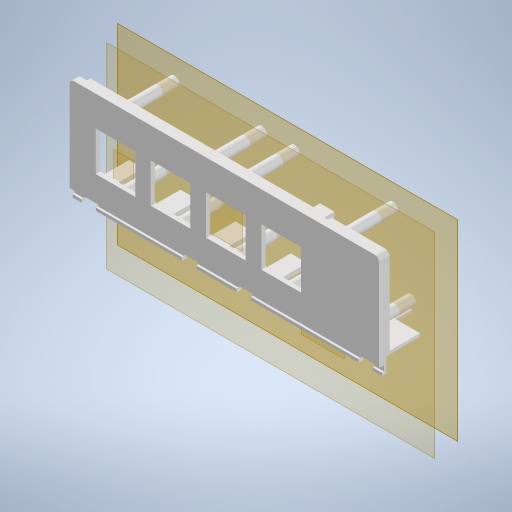
# Autodesk Inventor part: RV_ES_TopHV
Saved by Autodesk Inventor 2023.3 (Build 273359000, 359)
## iProperties
Created: 2023-08-06
Part Number: RV_ES_TopHV
Material: Generic
Document SubType Name: Modeling
Designer: atrus
Density: 1 g/cm^3
Appearance: Default
Mass: 78.5507 g
Surface Area: 462.891 cm^2
Volume: 78.5507 cm^3
Author: atrus
Autodesk Inventor part; units mm, degrees
ref_plane "YZ Plane" through (0, 0, 0) normal (1, 0, 0) x (0, 1, 0)
ref_plane "XZ Plane" through (0, 0, 0) normal (0, 1, 0) x (-1, 0, 0)
ref_plane "XY Plane" through (0, 0, 0) normal (0, 0, 1) x (1, 0, 0)
ref_plane "Work Plane1" through (160.7185, -7.942384, -39.091557) normal (0, 0, 1) x (1, 0, 0)
ref_plane "Bottom Case Offset" through (160.7185, -7.942384, -38.891557) normal (0, 0, 1) x (1, 0, 0)
sketch "Sketch1" plane through (0, 0, 0) normal (0, 0, 1) x (1, 0, 0)
  line L0 (0, 55.614096) -> (215.9, 55.614096)
  line L1 (215.9, 55.614096) -> (215.9, 121.724616)
  line L2 (215.9, 121.724616) -> (0, 121.724616)
  line L3 (0, 121.724616) -> (0, 55.614096)
  line L4 (215.9, 121.724616) -> (215.9, 57.656276) construction
  line L5 (0, 48.884616) -> (0, 118.549616)
  line L6 (1.113, 48.884616) -> (0, 48.884616)
  point P0 (0, 88.669356)
  constraints: 10 end point, 2 parallel, 1 horizontal, 1 midpoint, 1 perpendicular
extrude "Top Face" add sketch "Sketch1" along normal blind 5
sketch "Sketch2" plane through (0, 0, 5) normal (0, 0, 1) x (1, 0, 0)
  line L0 (44.754719, 74.175735) -> (19.253119, 74.175735) construction
  line L1 (44.754719, 99.677335) -> (44.754719, 74.175735) construction
  line L2 (19.253119, 74.175735) -> (19.253119, 99.677335) construction
  line L3 (57.607119, 74.175735) -> (57.607119, 99.677335) construction
  line L4 (83.108719, 99.677335) -> (83.108719, 74.175735) construction
  line L5 (83.108719, 74.175735) -> (57.607119, 74.175735) construction
  line L6 (96.215119, 74.175735) -> (96.215119, 99.677335) construction
  line L7 (121.716719, 99.677335) -> (121.716719, 74.175735) construction
  line L8 (134.823119, 74.175735) -> (134.823119, 99.677335) construction
  line L9 (160.324719, 99.677335) -> (160.324719, 74.175735) construction
  line L10 (160.324719, 74.175735) -> (134.823119, 74.175735) construction
  line L11 (19.253119, 99.677335) -> (44.754719, 99.677335) construction
  line L12 (57.607119, 99.677335) -> (83.108719, 99.677335) construction
  line L13 (96.215119, 99.677335) -> (121.716719, 99.677335) construction
  line L14 (134.823119, 99.677335) -> (160.324719, 99.677335) construction
  line L15 (18.253119, 100.677335) -> (18.253119, 73.175735)
  line L16 (18.253119, 73.175735) -> (45.754719, 73.175735)
  line L17 (45.754719, 73.175735) -> (45.754719, 100.677335)
  line L18 (45.754719, 100.677335) -> (18.253119, 100.677335)
  line L19 (56.607119, 100.677335) -> (56.607119, 73.175735)
  line L20 (56.607119, 73.175735) -> (84.108719, 73.175735)
  line L21 (84.108719, 73.175735) -> (84.108719, 100.677335)
  line L22 (84.108719, 100.677335) -> (56.607119, 100.677335)
  line L23 (121.716719, 74.175735) -> (96.215119, 74.175735) construction
  line L24 (96.215119, 74.175735) -> (96.215119, 99.677335)
  line L25 (95.215119, 100.677335) -> (95.215119, 73.175735)
  line L26 (95.215119, 73.175735) -> (122.716719, 73.175735)
  line L27 (122.716719, 73.175735) -> (122.716719, 100.677335)
  line L28 (122.716719, 100.677335) -> (95.215119, 100.677335)
  line L29 (133.823119, 100.677335) -> (133.823119, 73.175735)
  line L30 (133.823119, 73.175735) -> (161.324719, 73.175735)
  line L31 (161.324719, 73.175735) -> (161.324719, 100.677335)
  line L32 (161.324719, 100.677335) -> (133.823119, 100.677335)
  point P0 (0, 0)
  dimension "d96" = 1
  constraints: 32 end point, 3 parallel, 12 other
  measures "d96" distance between parallel lines of L18 L11
extrude "Recept Cutouts" cut sketch "Sketch2" against normal blind 3
sketch "Sketch3" plane through (0, 0, 0) normal (0, 0, -1) x (-1, 0, 0)
  circle A0 centre (-90.17, 112.834616) radius 3.750005 construction
  circle A1 centre (-181.61, 112.834616) radius 3.750005 construction
  circle A2 centre (-29.21, 112.834616) radius 3.550005
  circle A3 centre (-32.004, 65.844616) radius 3.550005
  circle A4 centre (-70.358, 65.844616) radius 3.550005
  circle A5 centre (-90.17, 112.834616) radius 3.550005
  circle A6 centre (-113.03, 112.834616) radius 3.550005
  circle A7 centre (-108.966, 65.844616) radius 3.550005
  circle A8 centre (-181.61, 112.834616) radius 3.550005
  circle A9 centre (-194.31, 63.304616) radius 3.550005
  circle A10 centre (-29.21, 112.834616) radius 3.81
  circle A11 centre (-32.004, 65.844616) radius 3.81
  circle A12 centre (-113.03, 112.834616) radius 3.81
  circle A13 centre (-70.358, 65.844616) radius 3.81
  circle A14 centre (-108.966, 65.844616) radius 3.81
  circle A15 centre (-194.31, 63.304616) radius 3.81
  circle A16 centre (-147.574, 65.844616) radius 3.750005
  circle A17 centre (-147.574, 65.844616) radius 3.550005
  point P0 (0, 0)
  dimension "d5" = 0.2
  constraints: 9 centre point, 8 equal radius, 7 coincident
  measures "d5" radial gap between concentric circles of A1 A8
extrude "Bosses" add sketch "Sketch3" along normal up to surface (38.891557 mm away) contours A2 | A3 | A4 | A5 | A6 | A7 | A8 | A9 | A17
ref_plane "PCB Plane Offset" through (103.01683, 55.15644, -27.328797) normal (0, 0, 1) x (1, 0, 0)
sketch "Sketch4" plane through (0, 0, 0) normal (0, 0, -1) x (-1, 0, 0)
  line L0 (-188.196091, 44.678615) -> (-188.196091, 97.078617) construction
  line L1 (-188.696091, 55.614096) -> (-212.089995, 55.614096)
  line L2 (-212.089995, 55.614096) -> (-212.089995, 57.846616)
  line L3 (-212.089995, 57.846616) -> (-188.696091, 57.846616)
  line L4 (-188.696091, 57.846616) -> (-188.696091, 55.614096)
  line L5 (-172.95, 57.946616) -> (-195.35, 57.946616)
  line L6 (-212.08999, -4.005394) -> (-212.09, 115.374616)
  line L7 (0, 55.614096) -> (-215.9, 55.614096)
  point P0 (0, 0)
  dimension "d8" = 0.5
  dimension "d109" = 0.1
  constraints: 8 end point, 3 perpendicular, 1 collinear, 1 horizontal
  measures "d8" distance between parallel lines of L0 L4
  measures "d109" distance between parallel lines of L5 L3
extrude "PS Side Tall Barrier" add sketch "Sketch4" along normal up to surface (27.328797 mm away)
sketch "Sketch5" plane through (212.089995, 57.846616, -27.328797) normal (0, 0, -1) x (-1, 0, 0)
  line L0 (23.393904, 0) -> (23.393904, -2.23252)
  line L1 (23.393904, 0) -> (0, 0)
  line L2 (23.393904, -2.23252) -> (16.939975, -2.23252)
  line L3 (16.939975, -2.23252) -> (16.939975, 0)
  line L4 (16.939975, 0) -> (23.393904, 0)
  line L5 (23.393904, 0) -> (23.393904, -2.23252)
  point P0 (212.089995, -57.846616)
  point P1 (16.739975, -2.8)
  dimension "d13" = 0.2
  constraints: 8 end point, 2 parallel, 1 horizontal, 1 perpendicular, 1 point on line, 1 other
  measures "d13" horizontal distance of point (16.74, -2.8) L2.end
extrude "PS Side Tall Barrier PCB" add sketch "Sketch5" along normal up to surface (11.56276 mm away)
sketch "Sketch6" plane through (0, 0, 0) normal (0, 0, -1) x (-1, 0, 0)
  arc A0 (-212.725, 121.724616) -> (-215.9, 118.549616) centre (-212.725, 118.549616) ccw construction
  arc A1 (-210.312, 119.311616) -> (-213.487, 116.136616) centre (-210.312, 116.136616) ccw construction
  line L0 (-213.487, 50.884616) -> (-213.487, 116.136616) construction
  line L1 (-210.312, 119.311616) -> (-172.72, 119.311616) construction
  line L2 (-162.72, 119.311616) -> (-5.588, 119.311616) construction
  arc A2 (-2.413, 116.136616) -> (-5.588, 119.311616) centre (-5.588, 116.136616) ccw construction
  line L3 (-2.413, 58.624616) -> (-2.413, 50.884616) construction
  line L4 (-213.287, 58.146616) -> (-213.287, 116.136616)
  arc A3 (-210.312, 119.111616) -> (-213.287, 116.136616) centre (-210.312, 116.136616) ccw
  line L5 (-210.312, 119.111616) -> (-172.72, 119.111616)
  line L6 (-162.72, 119.111616) -> (-5.588, 119.111616)
  arc A4 (-2.613, 116.136616) -> (-5.588, 119.111616) centre (-5.588, 116.136616) ccw
  line L7 (-2.613, 116.136616) -> (-2.613, 61.064616)
  line L8 (-211.287, 58.146616) -> (-211.287, 116.136616)
  arc A5 (-210.312, 117.111616) -> (-211.287, 116.136616) centre (-210.312, 116.136616) ccw
  arc A6 (-4.613, 116.136616) -> (-5.588, 117.111616) centre (-5.588, 116.136616) ccw
  line L9 (-4.613, 116.136616) -> (-4.613, 61.064616)
  line L10 (-211.287, 58.146616) -> (-213.287, 58.146616)
  line L11 (-4.613, 61.064616) -> (-2.613, 61.064616)
  line L12 (-162.72, 119.111616) -> (-162.72, 117.111616)
  line L13 (-172.72, 117.111616) -> (-172.72, 119.111616)
  circle A7 centre (-181.61, 112.834616) radius 3.550005
  line L14 (-178.059995, 112.834616) -> (-178.059995, 117.111616)
  circle A8 centre (-113.03, 112.834616) radius 3.550005
  line L15 (-116.580005, 112.834616) -> (-116.580005, 117.111616)
  line L16 (-109.479995, 112.834616) -> (-109.479995, 117.111616)
  circle A9 centre (-90.17, 112.834616) radius 3.550005
  line L17 (-93.720005, 112.834616) -> (-93.720005, 117.111616)
  line L18 (-86.619995, 112.834616) -> (-86.619995, 117.111616)
  circle A10 centre (-29.21, 112.834616) radius 3.550005
  line L19 (-32.760005, 112.834616) -> (-32.760005, 117.111616)
  line L20 (-25.659995, 112.834616) -> (-25.659995, 117.111616)
  circle A11 centre (-181.61, 112.834616) radius 3.550005
  circle A12 centre (-113.03, 112.834616) radius 3.550005
  line L21 (-185.160005, 112.834616) -> (-185.160005, 117.111616)
  line L22 (-210.312, 117.111616) -> (-185.160005, 117.111616)
  line L23 (-178.059995, 117.111616) -> (-172.72, 117.111616)
  line L24 (-162.72, 117.111616) -> (-116.580005, 117.111616)
  line L25 (-109.479995, 117.111616) -> (-93.720005, 117.111616)
  line L26 (-86.619995, 117.111616) -> (-32.760005, 117.111616)
  line L27 (-25.659995, 117.111616) -> (-5.588, 117.111616)
  line L28 (-195.15002, 57.846616) -> (-212.089995, 57.846616)
  line L29 (-3.81001, 60.764616) -> (-8.88109, 60.764616) construction
  line L30 (-188.696091, 57.846616) -> (-195.15002, 57.846616) construction
  point P0 (-212.287, 58.146616)
  dimension "d59" = 0.2
  dimension "d60" = 0.2
  dimension "d62" = 2
  dimension "d113" = 2
  dimension "d114" = 0.3
  dimension "d115" = 0.3
  constraints: 48 end point, 24 perpendicular, 15 point on circle, 8 collinear, 7 tangent, 4 centre point, 3 vertical, 2 horizontal, 2 parallel, 1 midpoint, 8 other
  measures "d59" distance between parallel lines of L2 L6
  measures "d60" distance between parallel lines of L0 L4
  measures "d62" distance of L13.start L5.end
  measures "d113" distance between parallel lines of L8 L4
  measures "d114" distance between parallel lines of L29 L11
  measures "d115" distance from line of L30 point (-212.287, 58.147)
extrude "Inner Lip" add sketch "Sketch6" along normal blind 5 contours L4 A3 L5 L13 L23 L14 A7 L21 L22 A5 L8 L10 | L6 A4 L7 L11 L9 A6 L27 L20 A10 L19 L26 L18 A9 L17 L25 L16 A8 L15 L24 L12
sketch "Sketch7" plane through (181.61, 112.834616, -38.891557) normal (0, 0, -1) x (-1, 0, 0)
  circle A0 centre (0, 0) radius 3.550005
  circle A1 centre (68.58, 0) radius 3.550005
  circle A2 centre (91.44, 0) radius 3.550005
  circle A3 centre (152.4, 0) radius 3.550005
  circle A4 centre (149.606, -46.99) radius 3.550005
  circle A5 centre (111.252, -46.99) radius 3.550005
  circle A6 centre (72.644, -46.99) radius 3.550005
  circle A7 centre (-12.7, -49.53) radius 3.550005
  circle A8 centre (34.036, -46.99) radius 3.550005
  point P0 (181.61, -112.834616)
hole "Boss Holes" at (181.61, 112.834616, -38.891557) at (113.03, 112.834616, -38.891557) at (90.17, 112.834616, -38.891557) at (29.21, 112.834616, -38.891557) at (32.004, 65.844616, -38.891557) at (70.358, 65.844616, -38.891557) at (108.966, 65.844616, -38.891557) at (194.31, 63.304616, -38.891557) at (147.574, 65.844616, -38.891557) direction (0, 0, 1) diameter 2.15646 depth 12.7 tip angle 118 thread size "4-40 UNC" class "2B" standard "ANSI Unified Screw Threads"
sketch "Sketch8" plane through (0, 0, 0) normal (0, 0, -1) x (-1, 0, 0)
  line L0 (-162.72, 117.111616) -> (-162.72, 121.724616)
  line L1 (-215.9, 121.724616) -> (0, 121.724616)
  line L2 (-172.72, 117.111616) -> (-172.72, 121.724616)
  line L3 (-162.72, 117.111616) -> (-116.580005, 117.111616) construction
  line L4 (-172.72, 117.111616) -> (-162.72, 117.111616)
  line L5 (-178.059995, 117.111616) -> (-172.72, 117.111616)
  line L6 (-172.72, 117.111616) -> (-172.72, 119.111616)
  line L7 (-162.72, 119.111616) -> (-162.72, 117.111616)
  line L8 (-172.72, 121.724616) -> (-162.72, 121.724616)
  point P0 (0, 0)
  point P1 (-172.72, 118.111616)
  constraints: 8 end point, 3 collinear, 1 horizontal, 1 midpoint, 1 perpendicular, 1 point on line, 1 vertical
extrude "Cord Relief" add sketch "Sketch8" along normal blind 7
fillet "Boss Filets" radius 3.175 9 edges at (181.61, 109.2846, 0) (35.554, 65.8446, 0) (73.908, 65.8446, 0) (112.516, 65.8446, 0) (197.86, 63.3046, 0) (113.03, 109.2846, 0) (90.17, 109.2846, 0) (29.21, 109.2846, 0) (151.124, 65.8446, 0)
ref_plane "Relay Top" through (28.37801, 48.104546, -10.841317) normal (0, 0, 1) x (0, -1, 0)
ref_plane "PS Top" through (155.310019, 43.098635, -2.554097) normal (0, 0, 1) x (0, 1, 0)
ref_plane "Work Plane7" through (-216.350226, -15.116245, -29.091557) normal (0, 0, 1) x (1, -0.0000001, 0)
sketch "Sketch10" plane through (0, 0, 0) normal (0, 0, -1) x (-1, 0, 0)
  line L0 (-160.996089, 97.078617) -> (-160.996089, 44.678615) construction
  line L1 (-188.196091, 44.678615) -> (-188.196091, 97.078617) construction
  line L2 (-122.08008, 67.154546) -> (-134.78008, 67.154546) construction
  line L3 (-134.78008, 67.154546) -> (-134.78008, 96.154546) construction
  line L4 (-134.78008, 96.154546) -> (-122.08008, 96.154546) construction
  line L5 (-122.08008, 96.154546) -> (-122.08008, 67.154546) construction
  line L6 (-123.43008, 68.054546) -> (-133.43008, 68.054546) construction
  line L7 (-123.43008, 69.054546) -> (-123.43008, 68.054546) construction
  line L8 (-133.43008, 69.054546) -> (-123.43008, 69.054546) construction
  line L9 (-133.43008, 68.054546) -> (-133.43008, 69.054546) construction
  line L10 (-133.83008, 88.254546) -> (-133.83008, 84.654546) construction
  line L11 (-133.83008, 84.654546) -> (-123.03008, 84.654546) construction
  line L12 (-123.03008, 84.654546) -> (-123.03008, 88.254546) construction
  line L13 (-123.03008, 88.254546) -> (-133.83008, 88.254546) construction
  line L14 (-83.21808, 67.154556) -> (-95.91808, 67.154556) construction
  line L15 (-95.91808, 67.154556) -> (-95.91808, 96.154556) construction
  line L16 (-95.91808, 96.154556) -> (-83.21808, 96.154556) construction
  line L17 (-83.21808, 96.154556) -> (-83.21808, 67.154556) construction
  line L18 (-84.56808, 68.054556) -> (-94.56808, 68.054556) construction
  line L19 (-84.56808, 69.054556) -> (-84.56808, 68.054556) construction
  line L20 (-94.56808, 69.054556) -> (-84.56808, 69.054556) construction
  line L21 (-94.56808, 68.054556) -> (-94.56808, 69.054556) construction
  line L22 (-94.96808, 88.254556) -> (-94.96808, 84.654556) construction
  line L23 (-94.96808, 84.654556) -> (-84.16808, 84.654556) construction
  line L24 (-84.16808, 84.654556) -> (-84.16808, 88.254556) construction
  line L25 (-84.16808, 88.254556) -> (-94.96808, 88.254556) construction
  line L26 (-44.86408, 67.154546) -> (-57.56408, 67.154546) construction
  line L27 (-57.56408, 67.154546) -> (-57.56408, 96.154546) construction
  line L28 (-57.56408, 96.154546) -> (-44.86408, 96.154546) construction
  line L29 (-44.86408, 96.154546) -> (-44.86408, 67.154546) construction
  line L30 (-46.21408, 68.054546) -> (-56.21408, 68.054546) construction
  line L31 (-46.21408, 69.054546) -> (-46.21408, 68.054546) construction
  line L32 (-56.21408, 69.054546) -> (-46.21408, 69.054546) construction
  line L33 (-56.21408, 68.054546) -> (-56.21408, 69.054546) construction
  line L34 (-56.61408, 88.254546) -> (-56.61408, 84.654546) construction
  line L35 (-56.61408, 84.654546) -> (-45.81408, 84.654546) construction
  line L36 (-45.81408, 84.654546) -> (-45.81408, 88.254546) construction
  line L37 (-45.81408, 88.254546) -> (-56.61408, 88.254546) construction
  line L38 (-6.13608, 67.154546) -> (-18.83608, 67.154546) construction
  line L39 (-18.83608, 67.154546) -> (-18.83608, 96.154546) construction
  line L40 (-18.83608, 96.154546) -> (-6.13608, 96.154546) construction
  line L41 (-6.13608, 96.154546) -> (-6.13608, 67.154546) construction
  line L42 (-7.48608, 68.054546) -> (-17.48608, 68.054546) construction
  line L43 (-7.48608, 69.054546) -> (-7.48608, 68.054546) construction
  line L44 (-17.48608, 69.054546) -> (-7.48608, 69.054546) construction
  line L45 (-17.48608, 68.054546) -> (-17.48608, 69.054546) construction
  line L46 (-17.88608, 88.254546) -> (-17.88608, 84.654546) construction
  line L47 (-17.88608, 84.654546) -> (-7.08608, 84.654546) construction
  line L48 (-7.08608, 84.654546) -> (-7.08608, 88.254546) construction
  line L49 (-7.08608, 88.254546) -> (-17.88608, 88.254546) construction
  line L50 (-195.15002, 55.614096) -> (-188.696091, 55.614096)
  line L51 (-188.696091, 55.614096) -> (-188.696091, 57.846616)
  line L52 (-188.696091, 57.846616) -> (-195.15002, 57.846616)
  line L53 (-195.15002, 57.846616) -> (-195.15002, 55.614096)
  line L54 (0, 55.614096) -> (-215.9, 55.614096)
  line L55 (-188.696091, 57.846616) -> (-195.15002, 57.846616)
  arc A0 (-43.204, 60.994616) -> (-43.204, 57.994616) centre (-43.204, 59.494616) ccw construction
  arc A1 (-59.158, 57.994616) -> (-59.158, 60.994616) centre (-59.158, 59.494616) ccw construction
  arc A2 (-81.558, 60.994616) -> (-81.558, 57.994616) centre (-81.558, 59.494616) ccw construction
  arc A3 (-97.766, 57.994616) -> (-97.766, 60.994616) centre (-97.766, 59.494616) ccw construction
  arc A4 (-120.166, 60.994616) -> (-120.166, 57.994616) centre (-120.166, 59.494616) ccw construction
  arc A5 (-135.358, 57.994616) -> (-135.358, 60.994616) centre (-135.358, 59.494616) ccw construction
  arc A6 (-157.758, 60.994616) -> (-157.758, 57.994616) centre (-157.758, 59.494616) ccw construction
  arc A7 (-20.804, 57.994616) -> (-20.804, 60.994616) centre (-20.804, 59.494616) ccw construction
  line L56 (-8.88109, 60.764616) -> (-8.88109, 58.224616) construction
  line L57 (-9.18109, 60.994616) -> (-19.004, 60.994616)
  line L58 (-19.004, 60.994616) -> (-19.004, 57.994616)
  line L59 (-19.004, 57.994616) -> (-9.18109, 57.994616)
  line L60 (-9.18109, 57.994616) -> (-9.18109, 60.994616)
  line L61 (-20.804, 57.994616) -> (-8.060378, 57.994616) construction
  line L62 (-20.804, 60.994616) -> (-8.354564, 60.994616) construction
  line L63 (-45.004, 60.994616) -> (-57.358, 60.994616)
  line L64 (-57.358, 60.994616) -> (-57.358, 57.994616)
  line L65 (-57.358, 57.994616) -> (-45.004, 57.994616)
  line L66 (-45.004, 57.994616) -> (-45.004, 60.994616)
  line L67 (-83.358, 57.994616) -> (-95.966, 57.994616)
  line L68 (-95.966, 57.994616) -> (-95.966, 60.994616)
  line L69 (-95.966, 60.994616) -> (-83.358, 60.994616)
  line L70 (-83.358, 60.994616) -> (-83.358, 57.994616)
  line L71 (-121.966, 57.994616) -> (-133.558, 57.994616)
  line L72 (-133.558, 57.994616) -> (-133.558, 60.994616)
  line L73 (-133.558, 60.994616) -> (-121.966, 60.994616)
  line L74 (-121.966, 60.994616) -> (-121.966, 57.994616)
  point P0 (-19.304, 59.494616)
  point P1 (-9.18109, 59.494616)
  point P2 (-45.004, 59.494616)
  point P3 (-44.704, 59.494616)
  point P4 (-57.658, 59.494616)
  point P5 (-57.358, 59.494616)
  point P6 (-83.358, 59.494616)
  point P7 (-83.058, 59.494616)
  point P8 (-96.266, 59.494616)
  point P9 (-95.966, 59.494616)
  point P10 (-121.666, 59.494616)
  point P11 (-121.966, 59.494616)
  point P12 (-133.858, 59.494616)
  point P13 (-133.558, 59.494616)
  dimension "d101" = 0.3
  dimension "d102" = 0.3
  dimension "d103" = 0.3
  dimension "d104" = 0.3
  dimension "d105" = 0.3
  dimension "d106" = 0.3
  dimension "d107" = 0.3
  dimension "d108" = 0.3
  constraints: 36 end point, 8 collinear, 8 parallel, 7 midpoint, 7 point on circle, 6 horizontal, 4 perpendicular
  measures "d101" distance from line of point (-19.304, 59.495) L58
  measures "d102" distance from line of point (-9.181, 59.495) L56
  measures "d103" distance of point (-45.004, 59.495) point (-44.704, 59.495)
  measures "d104" distance of point (-57.658, 59.495) point (-57.358, 59.495)
  measures "d105" distance of point (-83.358, 59.495) point (-83.058, 59.495)
  measures "d106" distance of point (-96.266, 59.495) point (-95.966, 59.495)
  measures "d107" distance of point (-121.666, 59.495) point (-121.966, 59.495)
  measures "d108" distance of point (-133.858, 59.495) point (-133.558, 59.495)
extrude "Barrier Relay" add sketch "Sketch10" along normal up to surface (27.328797 mm away) contours L60 L59 L58 L57 | L66 L65 L64 L63 | L67 L68 L69 L70 | L71 L72 L73 L74
sketch "Sketch11" plane through (0, 0, 0) normal (0, 0, -1) x (-1, 0, 0)
  line L0 (-160.996089, 97.078617) -> (-160.996089, 44.678615) construction
  line L1 (-188.196091, 44.678615) -> (-188.196091, 97.078617) construction
  line L2 (0, 55.614096) -> (-215.9, 55.614096)
  line L3 (-187.696091, 55.614096) -> (-161.496089, 55.614096)
  line L4 (-161.496089, 55.614096) -> (-161.496089, 57.846616)
  line L5 (-161.496089, 57.846616) -> (-187.696091, 57.846616)
  line L6 (-187.696091, 57.846616) -> (-187.696091, 55.614096)
  line L7 (-188.696091, 57.846616) -> (-195.15002, 57.846616) construction
  point P0 (0, 0)
  point P1 (-187.696091, 56.730356)
  point P2 (-161.496089, 56.730356)
  dimension "d55" = 0.5
  dimension "d56" = 0.5
  constraints: 8 end point, 2 midpoint, 2 parallel, 1 collinear, 1 horizontal, 1 perpendicular, 1 point on line
  measures "d55" distance from line of L1 point (-187.696, 56.73)
  measures "d56" distance from line of point (-161.496, 56.73) L0
extrude "Barrier PSU" add sketch "Sketch11" along normal up to surface (2.554097 mm away)
fillet "Outside corner fillets" radius 3.175 2 edges at (215.9, 121.7246, 2.5) (0, 121.7246, 2.5)
fillet "Outer Boss Fillets" radius 3.175 4 edges at (29.21, 116.3846, -5) (90.17, 116.3846, -5) (113.03, 116.3846, -5) (181.61, 116.3846, -5)
ref_plane "TopReceptSeatOffset" through (100.625339, 92.026755, 2.44) normal (0, 0, 1) x (-1, 0, 0)
sketch "Sketch12" plane through (0, 0, 0) normal (0, 0, -1) x (-1, 0, 0)
  line L0 (-20.408819, 71.369035) -> (-43.599019, 71.369035) construction
  arc A0 (-20.408819, 71.369035) -> (-16.446419, 75.331435) centre (-20.408819, 75.331435) ccw construction
  line L1 (-16.446419, 98.521635) -> (-16.446419, 75.331435) construction
  arc A1 (-16.446419, 98.521635) -> (-20.408819, 102.484035) centre (-20.408819, 98.521635) ccw construction
  line L2 (-43.599019, 102.484035) -> (-20.408819, 102.484035) construction
  arc A2 (-43.599019, 102.484035) -> (-47.561419, 98.521635) centre (-43.599019, 98.521635) ccw construction
  line L3 (-47.561419, 75.331435) -> (-47.561419, 98.521635) construction
  arc A3 (-47.561419, 75.331435) -> (-43.599019, 71.369035) centre (-43.599019, 75.331435) ccw construction
  line L4 (-43.167219, 74.975835) -> (-20.815219, 74.975835) construction
  arc A4 (-43.929219, 75.737835) -> (-43.167219, 74.975835) centre (-43.167219, 75.737835) ccw construction
  line L5 (-43.929219, 88.691835) -> (-43.929219, 75.737835) construction
  arc A5 (-43.167219, 89.453835) -> (-43.929219, 88.691835) centre (-43.167219, 88.691835) ccw construction
  line L6 (-40.385919, 89.453835) -> (-43.167219, 89.453835) construction
  arc A6 (-40.385919, 89.453835) -> (-39.623919, 90.215835) centre (-40.385919, 90.215835) ccw construction
  line L7 (-39.623919, 98.089835) -> (-39.623919, 90.215835) construction
  arc A7 (-38.861919, 98.851835) -> (-39.623919, 98.089835) centre (-38.861919, 98.089835) ccw construction
  line L8 (-25.145919, 98.851835) -> (-38.861919, 98.851835) construction
  arc A8 (-24.383919, 98.089835) -> (-25.145919, 98.851835) centre (-25.145919, 98.089835) ccw construction
  line L9 (-24.383919, 90.215835) -> (-24.383919, 98.089835) construction
  arc A9 (-24.383919, 90.215835) -> (-23.621919, 89.453835) centre (-23.621919, 90.215835) ccw construction
  line L10 (-20.815219, 89.453835) -> (-23.621919, 89.453835) construction
  arc A10 (-20.053219, 88.691835) -> (-20.815219, 89.453835) centre (-20.815219, 88.691835) ccw construction
  line L11 (-20.053219, 75.737835) -> (-20.053219, 88.691835) construction
  arc A11 (-20.815219, 74.975835) -> (-20.053219, 75.737835) centre (-20.815219, 75.737835) ccw construction
  line L12 (-58.762819, 71.369035) -> (-81.953019, 71.369035) construction
  arc A12 (-58.762819, 71.369035) -> (-54.800419, 75.331435) centre (-58.762819, 75.331435) ccw construction
  line L13 (-54.800419, 98.521635) -> (-54.800419, 75.331435) construction
  arc A13 (-54.800419, 98.521635) -> (-58.762819, 102.484035) centre (-58.762819, 98.521635) ccw construction
  line L14 (-81.953019, 102.484035) -> (-58.762819, 102.484035) construction
  arc A14 (-81.953019, 102.484035) -> (-85.915419, 98.521635) centre (-81.953019, 98.521635) ccw construction
  line L15 (-85.915419, 75.331435) -> (-85.915419, 98.521635) construction
  arc A15 (-85.915419, 75.331435) -> (-81.953019, 71.369035) centre (-81.953019, 75.331435) ccw construction
  line L16 (-81.521219, 74.975835) -> (-59.169219, 74.975835) construction
  arc A16 (-82.283219, 75.737835) -> (-81.521219, 74.975835) centre (-81.521219, 75.737835) ccw construction
  line L17 (-82.283219, 88.691835) -> (-82.283219, 75.737835) construction
  arc A17 (-81.521219, 89.453835) -> (-82.283219, 88.691835) centre (-81.521219, 88.691835) ccw construction
  line L18 (-78.739919, 89.453835) -> (-81.521219, 89.453835) construction
  arc A18 (-78.739919, 89.453835) -> (-77.977919, 90.215835) centre (-78.739919, 90.215835) ccw construction
  line L19 (-77.977919, 98.089835) -> (-77.977919, 90.215835) construction
  arc A19 (-77.215919, 98.851835) -> (-77.977919, 98.089835) centre (-77.215919, 98.089835) ccw construction
  line L20 (-63.499919, 98.851835) -> (-77.215919, 98.851835) construction
  arc A20 (-62.737919, 98.089835) -> (-63.499919, 98.851835) centre (-63.499919, 98.089835) ccw construction
  line L21 (-62.737919, 90.215835) -> (-62.737919, 98.089835) construction
  arc A21 (-62.737919, 90.215835) -> (-61.975919, 89.453835) centre (-61.975919, 90.215835) ccw construction
  line L22 (-59.169219, 89.453835) -> (-61.975919, 89.453835) construction
  arc A22 (-58.407219, 88.691835) -> (-59.169219, 89.453835) centre (-59.169219, 88.691835) ccw construction
  line L23 (-58.407219, 75.737835) -> (-58.407219, 88.691835) construction
  arc A23 (-59.169219, 74.975835) -> (-58.407219, 75.737835) centre (-59.169219, 75.737835) ccw construction
  line L24 (-124.523419, 75.331435) -> (-124.523419, 98.521635) construction
  arc A24 (-120.561019, 102.484035) -> (-124.523419, 98.521635) centre (-120.561019, 98.521635) ccw construction
  line L25 (-120.561019, 102.484035) -> (-97.370819, 102.484035) construction
  arc A25 (-93.408419, 98.521635) -> (-97.370819, 102.484035) centre (-97.370819, 98.521635) ccw construction
  line L26 (-93.408419, 98.521635) -> (-93.408419, 75.331435) construction
  arc A26 (-97.370819, 71.369035) -> (-93.408419, 75.331435) centre (-97.370819, 75.331435) ccw construction
  line L27 (-97.370819, 71.369035) -> (-120.561019, 71.369035) construction
  arc A27 (-124.523419, 75.331435) -> (-120.561019, 71.369035) centre (-120.561019, 75.331435) ccw construction
  line L28 (-96.215119, 74.175735) -> (-121.716719, 74.175735) construction
  line L29 (-96.215119, 99.677335) -> (-96.215119, 74.175735) construction
  line L30 (-121.716719, 99.677335) -> (-96.215119, 99.677335) construction
  line L31 (-121.716719, 74.175735) -> (-121.716719, 99.677335) construction
  line L32 (-135.978819, 71.369035) -> (-159.169019, 71.369035) construction
  arc A28 (-135.978819, 71.369035) -> (-132.016419, 75.331435) centre (-135.978819, 75.331435) ccw construction
  line L33 (-132.016419, 98.521635) -> (-132.016419, 75.331435) construction
  arc A29 (-132.016419, 98.521635) -> (-135.978819, 102.484035) centre (-135.978819, 98.521635) ccw construction
  line L34 (-159.169019, 102.484035) -> (-135.978819, 102.484035) construction
  arc A30 (-159.169019, 102.484035) -> (-163.131419, 98.521635) centre (-159.169019, 98.521635) ccw construction
  line L35 (-163.131419, 75.331435) -> (-163.131419, 98.521635) construction
  arc A31 (-163.131419, 75.331435) -> (-159.169019, 71.369035) centre (-159.169019, 75.331435) ccw construction
  arc A32 (-58.762819, 75.331415) -> (-58.762799, 75.331435) centre (-58.762819, 75.331435) ccw
  arc A33 (-81.953038, 75.331435) -> (-81.953019, 75.331415) centre (-81.953019, 75.331435) ccw
  arc A34 (-81.953019, 98.521654) -> (-81.953038, 98.521635) centre (-81.953019, 98.521635) ccw
  arc A35 (-58.762799, 98.521635) -> (-58.762819, 98.521654) centre (-58.762819, 98.521635) ccw
  arc A36 (-135.978819, 75.331239) -> (-135.978623, 75.331435) centre (-135.978819, 75.331435) ccw
  arc A37 (-159.169214, 75.331435) -> (-159.169019, 75.331239) centre (-159.169019, 75.331435) ccw
  arc A38 (-159.169019, 98.52183) -> (-159.169214, 98.521635) centre (-159.169019, 98.521635) ccw
  arc A39 (-135.978623, 98.521635) -> (-135.978819, 98.52183) centre (-135.978819, 98.521635) ccw
  arc A40 (-131.016419, 98.521635) -> (-135.978819, 103.484035) centre (-135.978819, 98.521635) ccw
  line L36 (-131.016419, 98.521635) -> (-131.016419, 75.331435)
  arc A41 (-135.978819, 70.369035) -> (-131.016419, 75.331435) centre (-135.978819, 75.331435) ccw
  line L37 (-135.978819, 70.369035) -> (-159.169019, 70.369035)
  arc A42 (-164.131419, 75.331435) -> (-159.169019, 70.369035) centre (-159.169019, 75.331435) ccw
  line L38 (-164.131419, 75.331435) -> (-164.131419, 98.521635)
  arc A43 (-159.169019, 103.484035) -> (-164.131419, 98.521635) centre (-159.169019, 98.521635) ccw
  line L39 (-159.169019, 103.484035) -> (-135.978819, 103.484035)
  line L40 (-97.370819, 103.484035) -> (-120.561019, 103.484035)
  arc A44 (-120.561019, 103.484035) -> (-125.523419, 98.521635) centre (-120.561019, 98.521635) ccw
  line L41 (-125.523419, 98.521635) -> (-125.523419, 75.331435)
  arc A45 (-125.523419, 75.331435) -> (-120.561019, 70.369035) centre (-120.561019, 75.331435) ccw
  line L42 (-120.561019, 70.369035) -> (-97.370819, 70.369035)
  arc A46 (-97.370819, 70.369035) -> (-92.408419, 75.331435) centre (-97.370819, 75.331435) ccw
  line L43 (-92.408419, 75.331435) -> (-92.408419, 98.521635)
  arc A47 (-92.408419, 98.521635) -> (-97.370819, 103.484035) centre (-97.370819, 98.521635) ccw
  arc A48 (-53.800419, 98.521635) -> (-58.762819, 103.484035) centre (-58.762819, 98.521635) ccw
  line L44 (-53.800419, 98.521635) -> (-53.800419, 75.331435)
  arc A49 (-58.762819, 70.369035) -> (-53.800419, 75.331435) centre (-58.762819, 75.331435) ccw
  line L45 (-58.762819, 70.369035) -> (-81.953019, 70.369035)
  arc A50 (-86.915419, 75.331435) -> (-81.953019, 70.369035) centre (-81.953019, 75.331435) ccw
  line L46 (-86.915419, 75.331435) -> (-86.915419, 98.521635)
  arc A51 (-81.953019, 103.484035) -> (-86.915419, 98.521635) centre (-81.953019, 98.521635) ccw
  line L47 (-81.953019, 103.484035) -> (-58.762819, 103.484035)
  arc A52 (-15.446419, 98.521635) -> (-20.408819, 103.484035) centre (-20.408819, 98.521635) ccw
  line L48 (-15.446419, 98.521635) -> (-15.446419, 75.331435)
  arc A53 (-20.408819, 70.369035) -> (-15.446419, 75.331435) centre (-20.408819, 75.331435) ccw
  line L49 (-20.408819, 70.369035) -> (-43.599019, 70.369035)
  arc A54 (-48.561419, 75.331435) -> (-43.599019, 70.369035) centre (-43.599019, 75.331435) ccw
  line L50 (-48.561419, 75.331435) -> (-48.561419, 98.521635)
  arc A55 (-43.599019, 103.484035) -> (-48.561419, 98.521635) centre (-43.599019, 98.521635) ccw
  line L51 (-43.599019, 103.484035) -> (-20.408819, 103.484035)
  point P0 (0, 0)
  dimension "d97" = 1
  dimension "d98" = 1
  dimension "d99" = 1
  dimension "d100" = 1
  constraints: 48 point on circle, 32 end point, 24 centre point, 28 other
  measures "d97" distance between parallel lines of L34 L39
  measures "d98" distance between parallel lines of L25 L40
  measures "d99" distance between parallel lines of L47 L14
  measures "d100" distance between parallel lines of L51 L2
extrude "Recept Inset" cut sketch "Sketch12" along normal blind 4 and the other way blind 2.0066 contours A36 | A37 | A38 | A39 | L36 A41 L37 A42 L38 A43 L39 A40 | A47 L43 A46 L42 A45 L41 A44 L40 | L44 A49 L45 A50 L46 A51 L47 A48 | L48 A53 L49 A54 L50 A55 L51 A52
sketch "Sketch13" plane through (0, 55.614096, 0) normal (-1, 0, 0) x (0, 0, 1)
  line L0 (0, 0) -> (-10.841317, 0)
  line L1 (0, 0) -> (5, 0)
  line L2 (0, 0) -> (5, 0)
  line L3 (0, -6.65) -> (0, 0)
  line L4 (0, 62.93552) -> (0, 0)
  line L5 (5, 0) -> (5, 62.93552)
  line L6 (5, 0) -> (5, 0)
  line L7 (4, -1) -> (1.5, -1)
  line L8 (1.5, -1) -> (1.5, -4.65)
  line L9 (1.5, -4.65) -> (3, -4.65)
  line L10 (3, -4.65) -> (3, -6.65)
  line L11 (3, -6.65) -> (0, -6.65)
  line L12 (5, 0) -> (4, -1)
  line L13 (-23.851557, -6.72948) -> (-0.1, -6.72948) construction
  line L14 (0, 0) -> (-10.841317, 0)
  line L15 (0, 0) -> (5, 0) construction
  line L16 (0, 0) -> (0, -7.071912) construction
  point P0 (0, -55.614096)
  point P1 (5, -1)
  point P2 (0, -3.325)
  point P3 (1.5, 0.07052)
  point P4 (1.5, 0)
  dimension "d73" = 2
  dimension "d74" = 1.5
  dimension "d75" = 1
  dimension "d77" = 1
  dimension "d78" = 1
  dimension "d110" = 2
  dimension "d111" = 3.65
  constraints: 24 end point, 5 perpendicular, 3 point on line, 2 vertical, 1 midpoint
  measures "d73" distance between parallel lines of L6 L10
  measures "d74" distance from line of point (0, -3.325) L8
  measures "d75" distance of L1.end point (5, -1)
  measures "d77" distance of L6.end point (5, -1)
  measures "d78" distance of L7.start point (5, -1)
  measures "d110" distance of L9.end L10.end
  measures "d111" distance of L7.end L8.end
extrude "TopFace Interlock" add sketch "Sketch13" against normal up to surface (215.9 mm away)
sketch "Sketch14" plane through (0, 0, 5) normal (0, 0, 1) x (1, 0, 0)
  line L0 (18.253119, 109.567335) -> (45.754719, 109.567335) construction
  line L1 (56.353119, 109.567335) -> (84.108719, 109.567335) construction
  line L2 (94.453119, 109.567335) -> (122.716719, 109.567335) construction
  line L3 (132.553119, 109.567335) -> (161.324719, 109.567335) construction
  line L4 (133.823119, 100.677335) -> (161.324719, 100.677335) construction
  line L5 (95.215119, 100.677335) -> (122.716719, 100.677335) construction
  line L6 (56.607119, 100.677335) -> (84.108719, 100.677335) construction
  line L7 (18.253119, 100.677335) -> (45.754719, 100.677335) construction
  line L8 (145.823686, 109.567335) -> (146.101356, 108.565901)
  line L9 (146.101356, 108.565901) -> (147.876625, 108.565901)
  line L10 (147.876625, 108.565901) -> (148.163399, 109.567335)
  line L11 (148.163399, 109.567335) -> (149.110209, 109.567335)
  line L12 (149.110209, 109.567335) -> (147.608058, 104.487334)
  line L13 (147.608058, 104.487334) -> (146.269779, 104.487334)
  line L14 (146.269779, 104.487334) -> (144.763076, 109.567335)
  line L15 (144.763076, 109.567335) -> (145.823686, 109.567335)
  line L16 (146.975334, 105.415937) -> (147.649026, 107.782962)
  line L17 (147.649026, 107.782962) -> (146.319851, 107.782962)
  line L18 (146.319851, 107.782962) -> (146.975334, 105.415937)
  line L19 (110.2737, 109.567335) -> (110.2737, 104.487334)
  line L20 (110.2737, 104.487334) -> (108.63499, 104.487334)
  spline S0 degree 2 poles (108.63499, 104.487334) (107.765564, 104.487334) (106.900689, 105.092747) (106.900689, 105.707263) knots 0 0 0 1 2 2 2
  spline S1 degree 2 poles (106.900689, 105.707263) (106.900689, 105.893894) (106.991729, 106.258051) (107.17836, 106.558481) (107.45603, 106.790632) (107.647213, 106.858911) knots 0 0 0 1 2 3 4 4 4
  spline S2 degree 2 poles (107.647213, 106.858911) (107.45603, 106.890775) (107.11008, 107.072854) (106.850618, 107.36418) (106.700402, 107.760202) (106.700402, 108.006008) knots 0 0 0 1 2 3 4 4 4
  spline S3 degree 2 poles (106.700402, 108.006008) (106.700402, 108.784395) (107.742804, 109.567335) (108.72603, 109.567335) knots 0 0 0 1 2 2 2
  line L21 (108.72603, 109.567335) -> (110.2737, 109.567335)
  spline S4 degree 2 poles (108.65775, 108.784395) (108.430152, 108.784395) (108.084202, 108.666044) (107.847499, 108.461205) (107.729148, 108.183535) (107.729148, 108.024216) knots 0 0 0 1 2 3 4 4 4
  spline S5 degree 2 poles (107.729148, 108.024216) (107.729148, 107.691922) (108.220761, 107.318661) (108.730582, 107.318661) knots 0 0 0 1 2 2 2
  line L22 (108.730582, 107.318661) -> (109.32689, 107.318661)
  line L23 (109.32689, 107.318661) -> (109.32689, 108.784395)
  line L24 (109.32689, 108.784395) -> (108.65775, 108.784395)
  spline S6 degree 2 poles (107.897571, 105.875686) (107.897571, 105.730023) (107.98861, 105.497872) (108.198001, 105.338553) (108.521191, 105.247514) (108.74879, 105.247514) knots 0 0 0 1 2 3 4 4 4
  line L25 (108.74879, 105.247514) -> (109.32689, 105.247514)
  line L26 (109.32689, 105.247514) -> (109.32689, 106.585793)
  line L27 (109.32689, 106.585793) -> (108.74879, 106.585793)
  spline S7 degree 2 poles (108.74879, 106.585793) (108.516639, 106.585793) (108.193449, 106.471994) (107.98861, 106.276259) (107.897571, 106.021349) (107.897571, 105.875686) knots 0 0 0 1 2 3 4 4 4
  spline S8 degree 2 poles (68.519377, 109.362496) (68.856223, 109.499055) (69.488947, 109.635614) (69.834897, 109.635614) knots 0 0 0 1 2 2 2
  spline S9 degree 2 poles (69.834897, 109.635614) (70.381134, 109.635614) (71.223248, 109.312424) (71.801349, 108.675148) (72.101779, 107.73289) (72.101779, 107.104718) knots 0 0 0 1 2 3 4 4 4
  spline S10 degree 2 poles (72.101779, 107.104718) (72.101779, 106.46289) (71.774037, 105.466008) (71.168625, 104.774109) (70.30375, 104.414503) (69.762066, 104.414503) knots 0 0 0 1 2 3 4 4 4
  spline S11 degree 2 poles (69.762066, 104.414503) (69.589091, 104.414503) (69.279557, 104.428159) (68.983679, 104.473678) (68.683248, 104.541958) (68.519377, 104.596582) knots 0 0 0 1 2 3 4 4 4
  line L28 (68.519377, 104.596582) -> (68.519377, 105.543392)
  spline S12 degree 2 poles (68.519377, 105.543392) (68.847119, 105.388625) (69.44798, 105.256618) (69.693786, 105.256618) knots 0 0 0 1 2 2 2
  spline S13 degree 2 poles (69.693786, 105.256618) (70.053392, 105.256618) (70.563213, 105.51608) (70.895507, 105.989485) (71.050274, 106.635865) (71.050274, 107.027334) knots 0 0 0 1 2 3 4 4 4
  spline S14 degree 2 poles (71.050274, 107.027334) (71.050274, 107.437012) (70.890955, 108.087944) (70.558661, 108.538589) (70.035184, 108.775291) (69.68013, 108.775291) knots 0 0 0 1 2 3 4 4 4
  spline S15 degree 2 poles (69.68013, 108.775291) (69.552675, 108.775291) (69.252245, 108.72522) (68.947263, 108.643284) (68.646833, 108.529485) (68.519377, 108.470309) knots 0 0 0 1 2 3 4 4 4
  line L29 (68.519377, 108.470309) -> (68.519377, 109.362496)
  spline S16 degree 2 poles (30.028363, 106.963607) (30.028363, 107.555363) (30.319689, 108.515829) (30.938757, 109.198625) (31.899223, 109.567335) (32.572915, 109.567335) knots 0 0 0 1 2 3 4 4 4
  line L30 (32.572915, 109.567335) -> (33.861123, 109.567335)
  line L31 (33.861123, 109.567335) -> (33.861123, 104.487334)
  line L32 (33.861123, 104.487334) -> (32.358972, 104.487334)
  spline S17 degree 2 poles (32.358972, 104.487334) (31.77632, 104.487334) (30.902342, 104.778661) (30.319689, 105.384073) (30.028363, 106.317227) (30.028363, 106.963607) knots 0 0 0 1 2 3 4 4 4
  spline S18 degree 2 poles (31.052557, 107.027334) (31.052557, 106.613105) (31.184564, 105.966725) (31.49865, 105.520632) (32.026679, 105.288481) (32.418148, 105.288481) knots 0 0 0 1 2 3 4 4 4
  line L33 (32.418148, 105.288481) -> (32.905209, 105.288481)
  line L34 (32.905209, 105.288481) -> (32.905209, 108.766188)
  line L35 (32.905209, 108.766188) -> (32.486428, 108.766188)
  spline S19 degree 2 poles (32.486428, 108.766188) (31.780872, 108.766188) (31.052557, 107.928625) (31.052557, 107.027334) knots 0 0 0 1 2 2 2
  point P0 (0, 0)
  dimension "d112" = 8.89
  constraints: 8 end point, 4 horizontal, 4 vertical alignment, 3 collinear
  measures "d112" distance between parallel lines of L4 L3
extrude "Extrusion13" cut sketch "Sketch14" against normal blind 0.001
sketch "Sketch16" plane through (0, 0, 0) normal (0, 0, -1) x (-1, 0, 0)
  circle A0 centre (-204.47, 50.604616) radius 3.450005 construction
  circle A1 centre (-204.47, 50.604616) radius 4.99402
  line L0 (-212.089995, 55.598636) -> (-188.696091, 55.598636)
  circle A2 centre (-119.38, 50.604616) radius 3.450005 construction
  circle A3 centre (-81.28, 50.604616) radius 3.450005 construction
  circle A4 centre (-11.43, 50.604616) radius 3.450005 construction
  circle A5 centre (-119.38, 50.604616) radius 5.00948
  line L1 (0, 55.614096) -> (-215.9, 55.614096) construction
  circle A6 centre (-81.28, 50.604616) radius 5.00948
  circle A7 centre (-11.43, 50.604616) radius 5.00948
  point P0 (0, 0)
  constraints: 4 centre point, 4 coincident, 4 tangent
extrude "Extrusion14" cut sketch "Sketch16" against normal blind 25.4
equation "\"d78\" = d77"
body "Solid1"
